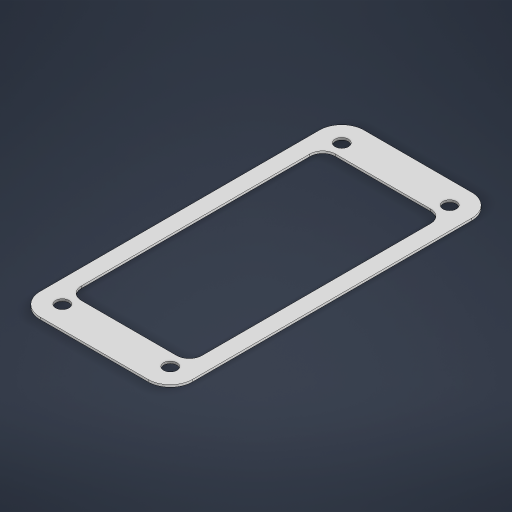
# Autodesk Inventor part: GearBoxSpacers
Saved by Autodesk Inventor 2024 (Build 280153000, 153)
## iProperties
Created: 2024-02-26
Part Number: GearBoxSpacers
Material: Generic
Document SubType Name: Modeling
Designer: avsar
Density: 1 g/cm^3
Appearance: Default
Author: avsar
Autodesk Inventor part; units mm, degrees
ref_plane "YZ Plane" through (0, 0, 0) normal (1, 0, 0) x (0, 1, 0)
ref_plane "XZ Plane" through (0, 0, 0) normal (0, 1, 0) x (-1, 0, 0)
ref_plane "XY Plane" through (0, 0, 0) normal (0, 0, 1) x (1, 0, 0)
sketch "Sketch1" plane through (0, 0, 0) normal (0, 1, 0) x (-1, 0, 0)
  line L0 (24, 51) -> (-24, 51)
  line L1 (-24, 51) -> (-24, -51)
  line L2 (-24, -51) -> (24, -51)
  line L3 (24, -51) -> (24, 51)
  line L4 (24, 51) -> (-24, -51) construction
  line L5 (-24, 51) -> (24, -51) construction
  point P0 (0, 0)
  dimension "d0" = 48
  dimension "d1" = 102
  constraints: 12 end point, 2 midpoint, 2 parallel, 1 horizontal, 1 perpendicular
  measures "d0" distance of L2.end L1.end
  measures "d1" distance of L1.end L0.end
extrude "Extrusion1" add sketch "Sketch1" along normal blind 0.7
fillet "Fillet1" radius 7 4 edges at (-24, 0.35, 51) (24, 0.35, 51) (24, 0.35, -51) (-24, 0.35, -51)
sketch "Sketch2" plane through (0, 0.7, 0) normal (0, 1, 0) x (1, 0, 0)
  circle A0 centre (-17, 44) radius 2.1
  arc A1 (-17, 51) -> (-24, 44) centre (-17, 44) ccw construction
  circle A2 centre (17, 44) radius 2.1
  arc A3 (24, 44) -> (17, 51) centre (17, 44) ccw construction
  circle A4 centre (-17, -44) radius 2.1
  arc A5 (-24, -44) -> (-17, -51) centre (-17, -44) ccw construction
  circle A6 centre (17, -44) radius 2.1
  arc A7 (17, -51) -> (24, -44) centre (17, -44) ccw construction
  point P0 (0, 0)
  dimension "d5" = 4.2
  dimension "d6" = 4.2
  dimension "d7" = 4.2
  dimension "d8" = 4.2
  constraints: 4 centre point, 4 concentric
  measures "d5" diameter of A0
  measures "d6" diameter of A2
  measures "d7" diameter of A4
  measures "d8" diameter of A6
extrude "Extrusion2" cut sketch "Sketch2" against normal through all
sketch "Sketch3" plane through (0, 0.7, 0) normal (0, 1, 0) x (1, 0, 0)
  line L0 (-19, -40) -> (19, -40)
  line L1 (19, -40) -> (19, 40)
  line L2 (19, 40) -> (-19, 40)
  line L3 (-19, 40) -> (-19, -40)
  line L4 (-19, -40) -> (19, 40) construction
  line L5 (19, -40) -> (-19, 40) construction
  point P0 (0, 0)
  dimension "d11" = 38
  dimension "d12" = 80
  constraints: 12 end point, 2 midpoint, 2 parallel, 1 horizontal, 1 perpendicular
  measures "d11" distance of L2.end L1.end
  measures "d12" distance of L1.end L0.end
extrude "Extrusion3" cut sketch "Sketch3" against normal through all
fillet "Fillet2" radius 4 4 edges at (-19, 0.35, -40) (19, 0.35, -40) (19, 0.35, 40) (-19, 0.35, 40)
body "Solid1"
